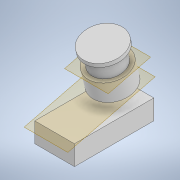
# Autodesk Inventor part: HGT
Saved by Autodesk Inventor 2022 (Build 260153000, 153)
## iProperties
Created: 2022-12-05
Part Number: HGT
Material: Generic
Document SubType Name: Modeling
Designer: nguye
Density: 1 g/cm^3
Appearance: Default
Author: nguye
Autodesk Inventor part; units mm, degrees
ref_plane "YZ Plane" through (0, 0, 0) normal (1, 0, 0) x (0, 1, 0)
ref_plane "XZ Plane" through (0, 0, 0) normal (0, 1, 0) x (-1, 0, 0)
ref_plane "XY Plane" through (0, 0, 0) normal (0, 0, 1) x (1, 0, 0)
sketch "Sketch1" plane through (0, 0, 0) normal (1, 0, 0) x (0, 1, 0)
  point P0 (0, 0)
sketch "Sketch2" plane through (0, 0, 0) normal (0, 1, 0) x (-1, 0, 0)
  line L0 (5, -10) -> (-5, -10)
  line L1 (-5, -10) -> (-5, 10)
  line L2 (-5, 10) -> (5, 10)
  line L3 (5, 10) -> (5, -10)
  line L4 (5, -10) -> (-5, 10) construction
  line L5 (-5, -10) -> (5, 10) construction
  point P0 (0, 0)
  dimension "d0" = 10
  dimension "d1" = 20
  constraints: 12 end point, 2 midpoint, 2 parallel, 1 horizontal, 1 perpendicular
  measures "d0" distance of L1.end L2.end
  measures "d1" distance of L0.end L1.end
extrude "Extrusion1" add sketch "Sketch2" along normal blind 5
ref_plane "Work Plane2" through (-5, 5, 10) normal (0, 0.9702957, 0.2419219) x (1, 0, 0)
sketch "Sketch3" plane through (-5, 5, 10) normal (0, 0.9702957, 0.2419219) x (1, 0, 0)
  circle A0 centre (5, 15) radius 5
  line L0 (0, 0) -> (10, 0) projected
  point P0 (5, 8.4933)
  point P1 (5, 0)
  dimension "d6" = 10
  dimension "d7" = 15
  constraints: 1 centre point, 1 midpoint, 1 vertical alignment
  measures "d6" diameter of A0
  measures "d7" distance from line of A0.centre L0
extrude "Extrusion2" add sketch "Sketch3" along normal blind 10
ref_plane "Work Plane3" through (0, 13.4803, -3.3448) normal (0, 0.9702957, 0.2419219) x (1, 0, 0)
sketch "Sketch4" plane through (0, 13.4803, -3.3448) normal (0, 0.9702957, 0.2419219) x (1, 0, 0)
  circle A0 centre (0, 0) radius 5
  circle A1 centre (0, 0) radius 4
  point P0 (0, -6.5067)
  dimension "d11" = 8
  constraints: 2 centre point, 1 coincident
  measures "d11" diameter of A1
extrude "Extrusion3" cut sketch "Sketch4" along normal blind 4
equation "\"d8\" = d6"
body "Solid1"
